inertial_disk (Autodesk Fusion 360 design; units mm, degrees)
part number: 2026-10-07-20-45-40-601
Autodesk Fusion 360 part; units mm, degrees
sketch "Sketch1" plane through (0, 0, 0) normal (0, 0, 1) x (1, 0, 0)
  circle A0 centre (0, 0) radius 4.1
  circle A1 centre (0, 0) radius 35
  circle A2 centre (0, 0) radius 8 construction
  circle A3 centre (0, 0) radius 25 construction
  circle A4 centre (0, 25) radius 6.3
  circle A5 centre (0, 25) radius 3.2
  circle A6 centre (0, 8) radius 1.6
  circle A7 centre (-6.9282, -4) radius 1.6
  circle A8 centre (6.9282, -4) radius 1.6
  circle A9 centre (-17.6777, 17.6777) radius 3.2
  circle A10 centre (-25, 0) radius 3.2
  circle A11 centre (-17.6777, -17.6777) radius 3.2
  circle A12 centre (0, -25) radius 3.2
  circle A13 centre (17.6777, -17.6777) radius 3.2
  circle A14 centre (25, 0) radius 3.2
  circle A15 centre (17.6777, 17.6777) radius 3.2
  dimension "d1" = 8.2
  dimension "d2" = 50
  dimension "d3" = 70
  dimension "d4" = 16
  dimension "d5" = 12.6
  dimension "d6" = 6.4
  dimension "d7" = 3.2
  dimension "d9" = 360
  dimension "d11" = 360
  constraint coincident A0.centre A1.centre
  constraint concentric A0 A2
  constraint concentric A2 A3
  constraint coincident A3 A4.centre
  constraint concentric A4 A5
  constraint coincident A2 A6.centre
  measures "d1" diameter of A0
  measures "d2" diameter of A3
  measures "d3" diameter of A1
  measures "d4" diameter of A2
  measures "d5" diameter of A4
  measures "d6" diameter of A5
  measures "d7" diameter of A6
extrude "Extrude1" add sketch "Sketch1" along normal blind 6 contours A1 | A4
